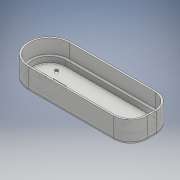
# Autodesk Inventor part: top
Saved by Autodesk Inventor 2017 (Build 210142000, 142)
## iProperties
Part Number: top
Material: Типовые
Document SubType Name: Modeling
Designer: roman
Density: 1 g/cm^3
Appearance: По умолчанию
Author: roman
Autodesk Inventor part; units mm, degrees
ref_plane "YZ Plane" through (0, 0, 0) normal (1, 0, 0) x (0, 1, 0)
ref_plane "XZ Plane" through (0, 0, 0) normal (0, 1, 0) x (-1, 0, 0)
ref_plane "XY Plane" through (0, 0, 0) normal (0, 0, 1) x (1, 0, 0)
sketch "Эскиз1" plane through (0, 0, 0) normal (0, 0, 1) x (1, 0, 0)
  arc A0 (37.9034, -0.2173) -> (42.261, 4.1403) centre (37.9034, 4.1403) ccw
  arc A1 (42.261, 8.15) -> (38.0283, 12.3827) centre (38.0283, 8.15) ccw
  arc A2 (43.261, 7.6552) -> (37.7725, 13.3827) centre (37.5283, 7.6552) ccw
  arc A3 (37.765, -1.2173) -> (43.261, 4.5105) centre (37.5283, 4.5105) ccw
  line L0 (37.765, -1.2173) -> (6.1001, -1.2173)
  line L1 (5.7034, -0.2173) -> (37.9034, -0.2173)
  line L2 (5.8283, 12.3827) -> (5.7034, -0.2173) construction
  arc A4 (5.8283, 12.3827) -> (5.7034, -0.2173) centre (6.0021, 6.0803) ccw
  arc A5 (6.1001, 13.3827) -> (6.1001, -1.2173) centre (6.1001, 6.0827) ccw
  line L3 (5.8283, 12.3827) -> (38.0283, 12.3827)
  line L4 (5.8283, 12.3827) -> (18.4289, 12.3827) construction
  line L5 (37.7725, 13.3827) -> (6.1001, 13.3827)
  line L6 (42.261, 8.15) -> (42.261, 4.1403)
  line L7 (43.261, 7.6552) -> (43.261, 4.5105)
  point P0 (0, 0)
  point P1 (0, 0)
  point P2 (0, 0)
  dimension "d10" = 1.5
  dimension "d0" = 90.568
  dimension "d1" = 4.2327
  dimension "d2" = 5.7327
  dimension "d3" = 5.7327
  dimension "d4" = 1
  dimension "d5" = 1
  dimension "d6" = 12.6
  dimension "d7" = 32.2
  dimension "d8" = 32.2
  dimension "d9" = 1
  constraints: 16 end point, 12 point on circle, 6 centre point, 6 tangent, 2 horizontal, 2 parallel, 2 vertical, 1 equal length
  measures "d0" angle of L2 L4
  measures "d1" radius of A1
  measures "d2" radius of A2
  measures "d3" radius of A3
  measures "d4" distance between parallel lines of L3 L5
  measures "d5" distance between parallel lines of L0 L1
  measures "d6" distance between parallel lines of L1 L3
  measures "d7" distance of L3.start L3.end
  measures "d8" distance of L1.start L1.end
  measures "d9" distance between parallel lines of L7 L6
extrude "main_walls" add sketch "Эскиз1" along normal blind 2
sketch "Эскиз2" plane through (0, 0, 0) normal (0, 0, -1) x (-1, 0, 0)
  line L0 (-6.1001, 13.3827) -> (-37.7725, 13.3827) projected
  arc A0 (-37.7725, 13.3827) -> (-43.261, 7.6552) centre (-37.5283, 7.6552) ccw projected
  line L1 (-43.261, 7.6552) -> (-43.261, 4.5105) projected
  arc A1 (-43.261, 4.5105) -> (-37.765, -1.2173) centre (-37.5283, 4.5105) ccw projected
  line L2 (-37.765, -1.2173) -> (-6.1001, -1.2173) projected
  arc A2 (-6.1001, -1.2173) -> (-6.1001, 13.3827) centre (-6.1001, 6.0827) ccw projected
  point P0 (0, 0)
extrude "top" add sketch "Эскиз2" along normal blind 0.8
sketch "Эскиз3" plane through (0, 0, -0.8) normal (0, 0, -1) x (-1, 0, 0)
  line L0 (-6.1001, 13.3827) -> (-37.7725, 13.3827) projected
  arc A0 (-37.7725, 13.3827) -> (-43.261, 7.6552) centre (-37.5283, 7.6552) ccw projected
  line L1 (-43.261, 7.6552) -> (-43.261, 4.5105) projected
  arc A1 (-43.261, 4.5105) -> (-37.765, -1.2173) centre (-37.5283, 4.5105) ccw projected
  line L2 (-37.765, -1.2173) -> (-6.1001, -1.2173) projected
  arc A2 (-6.1001, -1.2173) -> (-6.1001, 13.3827) centre (-6.1001, 6.0827) ccw projected
  line L3 (1.1999, -1.8994) -> (1.1999, 13.1826)
  line L4 (-7.4001, 0.4827) -> (-12.1001, 0.4827)
  line L5 (-12.1001, 0.4827) -> (-12.1001, 6.1827)
  line L6 (-12.1001, 6.1827) -> (-7.4001, 6.1827)
  line L7 (-7.4001, 6.1827) -> (-7.4001, 0.4827)
  circle A3 centre (-4.6001, 5.0827) radius 1
  circle A4 centre (-5.4001, 9.3827) radius 0.6
  line L8 (-33.761, 4.8827) -> (-35.261, 4.8827)
  line L9 (-35.261, 4.8827) -> (-35.261, 6.8827)
  line L10 (-35.261, 6.8827) -> (-33.761, 6.8827)
  line L11 (-33.761, 6.8827) -> (-33.761, 4.8827)
  point P0 (0, 0)
  dimension "d15" = 4.7
  dimension "d16" = 5.7
  dimension "d17" = 1.7
  dimension "d18" = 2
  dimension "d19" = 1.2
  dimension "d20" = 5.8
  dimension "d21" = 2.8
  dimension "d22" = 6.3
  dimension "d23" = 4
  dimension "d24" = 0.8
  dimension "d25" = 1.5
  dimension "d26" = 2
  dimension "d27" = 6.1
  dimension "d28" = 8
  constraints: 18 end point, 4 parallel, 2 centre point, 2 horizontal, 2 perpendicular, 1 tangent, 1 vertical
  measures "d15" distance of L5.end L6.end
  measures "d16" distance of L4.end L5.end
  measures "d17" distance between parallel lines of L4 L2
  measures "d18" diameter of A3
  measures "d19" diameter of A4
  measures "d20" distance from line of L3 A3.centre
  measures "d21" distance from line of A3.centre L7
  measures "d22" distance from line of L2 A3.centre
  measures "d23" distance from line of L0 A4.centre
  measures "d24" horizontal distance of A4.centre A3.centre
  measures "d25" distance of L9.end L10.end
  measures "d26" distance of L8.end L9.end
  measures "d27" distance between parallel lines of L8 L2
  measures "d28" distance between parallel lines of L1 L9
extrude "Выдавливание5" cut sketch "Эскиз3" against normal blind 1.8 contours L4 L5 L6 L7 | A3 | A4 | L8 L9 L10 L11
sketch "Эскиз8" plane through (0, 0, -0.8) normal (0, 0, -1) x (-1, 0, 0)
  line L0 (-33.761, 6.8827) -> (-33.761, 4.8827) projected
  line L1 (-33.761, 4.8827) -> (-35.261, 4.8827) projected
  line L2 (-35.261, 4.8827) -> (-35.261, 6.8827) projected
  line L3 (-35.261, 6.8827) -> (-33.761, 6.8827) projected
  circle A0 centre (-4.6001, 5.0827) radius 1 projected
  circle A1 centre (-5.4001, 9.3827) radius 0.6 projected
  line L4 (-7.4001, 6.1827) -> (-7.4001, 0.4827) projected
  line L5 (-7.4001, 0.4827) -> (-12.1001, 0.4827) projected
  line L6 (-12.1001, 0.4827) -> (-12.1001, 6.1827) projected
  line L7 (-12.1001, 6.1827) -> (-7.4001, 6.1827) projected
  line L8 (-6.1001, 13.3827) -> (-37.7725, 13.3827) projected
  arc A2 (-37.7725, 13.3827) -> (-43.261, 7.6552) centre (-37.5283, 7.6552) ccw projected
  line L9 (-43.261, 7.6552) -> (-43.261, 4.5105) projected
  arc A3 (-43.261, 4.5105) -> (-37.765, -1.2173) centre (-37.5283, 4.5105) ccw projected
  line L10 (-37.765, -1.2173) -> (-6.1001, -1.2173) projected
  arc A4 (-6.1001, -1.2173) -> (-6.1001, 13.3827) centre (-6.1001, 6.0827) ccw projected
  arc A5 (-6.1001, -1.8173) -> (-6.1001, 13.9827) centre (-6.1001, 6.0827) ccw
  line L11 (-6.1001, 13.9827) -> (-37.7813, 13.9827)
  line L12 (-6.1001, -1.8173) -> (-37.7733, -1.8173)
  arc A6 (-43.8609, 4.5105) -> (-37.7733, -1.8173) centre (-37.5283, 4.5105) ccw
  arc A7 (-37.7813, 13.9827) -> (-43.8609, 7.6552) centre (-37.5283, 7.6552) ccw
  line L13 (-43.8609, 7.6552) -> (-43.8609, 4.5105)
  point P0 (0, 0)
  dimension "d73" = 7.3
  dimension "d74" = 7.9
  constraints: 6 end point, 6 point on circle, 3 centre point, 3 coincident, 2 horizontal, 2 tangent, 1 vertical
  measures "d73" radius of A4
  measures "d74" radius of A5
extrude "Выдавливание8" add sketch "Эскиз8" against normal blind 8 contours L12 A6 L13 A7 L11 A5
fillet "Сопряжение3" radius 1 6 edges at (-1.7999, 6.0827, -0.8) (21.9407, 13.9827, -0.8) (21.9367, -1.8173, -0.8) (42.0919, 0.1202, -0.8) (42.0947, 12.0426, -0.8) (43.8609, 6.0828, -0.8)
equation "\"d2\" = d1 + d10"
equation "\"d3\" = d1 + d10"
equation "\"d5\" = d4"
equation "\"d7\" = d8"
equation "\"d9\" = d4"
